Autodesk Inventor part; units mm, degrees
note: some values were not read from the file. Chosen so that the rebuilt part matches the saved one: direction of "Hole1"; direction of "Hole2".
(part 2 of 2)
sketch "Sketch23" plane through (-31.8897, 11.2835, 1.2) normal (0, 1, 0) x (1, 0, 0)
  spline S0 degree 3 poles (23.3423, 2.1773) (22.9361, 2.2868) (22.2348, 2.4758) (21.6643, 2.8122) (20.9702, 2.8356) (21.0959, 3.0801) (21.2357, 3.2556) (21.545, 3.6296) (22.0063, 4.1628) (22.2757, 4.6965) (22.7863, 5.1713) (22.4442, 5.3817) (22.141, 5.5963) (20.9793, 6.2853) (19.3097, 7.5226) (17.5595, 9.6465) (16.7918, 11.5742) (16.5566, 12.9888) (16.5569, 13.9187) (16.7809, 15.2775) (17.4991, 17.0874) (19.0032, 19.0617) (20.3636, 20.2269) (21.2697, 20.7719) (21.4294, 20.8993) (21.6261, 20.977) (21.4367, 21.2372) (21.2991, 21.56) (20.9903, 22.0433) (20.7038, 22.5269) (20.5306, 22.8626) (20.3527, 23.2142) (21.0187, 23.2936) (21.6089, 23.6536) (22.2816, 23.8828) (22.6704, 24.0153) knots 0 0 0 0 0.120251 0.207576 0.243092 0.253486 0.278932 0.314291 0.397791 0.481584 0.525055 0.542669 0.585382 0.644073 0.940951 1.209833 1.457149 1.553131 1.638804 1.734787 1.964951 2.214573 2.471025 2.502064 2.525764 2.536995 2.553986 2.597546 2.658422 2.719524 2.763708 2.781717 2.817624 2.904325 3.023078 3.023078 3.023078 3.023078
  line L0 (22.6704, 24.0153) -> (24.8571, 24.8395)
  line L1 (24.8571, 24.8395) -> (25.7117, 23.9446)
  line L2 (25.7117, 23.9446) -> (26.5664, 23.0497)
  line L3 (26.5664, 23.0497) -> (27.2264, 23.2249)
  spline S1 degree 3 poles (27.2264, 23.2249) (28.1214, 23.3942) (30.0601, 23.7608) (33.0033, 23.8407) (35.2391, 23.7446) (36.5812, 23.5025) (37.0345, 23.4774) (37.3791, 23.3665) (37.6145, 23.6266) (37.901, 23.9483) (38.2952, 24.4873) (38.6552, 24.9486) (38.9707, 25.3794) (39.3411, 25.3443) (39.7891, 25.1189) (40.555, 24.8644) (41.485, 24.483) (42.4572, 24.1727) (43.0299, 23.8169) (43.5284, 23.7887) (43.5573, 23.623) (43.5154, 23.5368) (43.3485, 23.2629) (42.9997, 22.7627) (42.8221, 22.2309) (42.3636, 21.7129) (42.6831, 21.5669) (42.9326, 21.3965) (43.4921, 21.0841) (44.2214, 20.6257) (45.0881, 20.0008) (45.6191, 19.5378) (45.8847, 19.3063) knots 0 0 0 0 0.27293 0.59117 0.879686 0.945407 0.996033 1.020616 1.042904 1.091245 1.155662 1.23829 1.276828 1.298799 1.342169 1.428477 1.539037 1.646645 1.725219 1.757766 1.763106 1.772735 1.785452 1.860503 1.945316 1.986613 2.00195 2.036474 2.082721 2.190949 2.296581 2.40228 2.40228 2.40228 2.40228
  line L4 (45.8847, 19.3063) -> (46.4831, 18.7637)
  line L5 (46.4831, 18.7637) -> (45.5703, 17.7587)
  spline S2 degree 3 poles (45.5703, 17.7587) (45.3819, 17.552) (44.9926, 17.1246) (44.4311, 16.5127) (44.0571, 16.1085) (43.8856, 15.9233) knots 0 0 0 0 0.336837 0.696095 1 1 1 1
  line L6 (43.8856, 15.9233) -> (43.1137, 15.0928)
  line L7 (43.1137, 15.0928) -> (42.5787, 15.6278)
  spline S3 degree 3 poles (42.5787, 15.6278) (42.3692, 15.8216) (41.9418, 16.2171) (41.4347, 16.5497) (40.7785, 17.1236) (40.7564, 16.0848) (40.6522, 15.2342) (40.6358, 13.8016) (40.695, 12.2687) (40.9149, 11.2921) (40.9213, 9.8853) (41.7084, 10.5187) (42.2359, 10.931) (42.7621, 11.4456) (43.0392, 11.7879) (43.1734, 11.9381) (43.6929, 12.1595) (44.4272, 10.4542) (45.2768, 9.6626) (46.909, 8.4425) (45.7357, 7.4784) (44.7926, 6.6607) (43.8619, 6.074) (43.3923, 5.7779) knots 0 0 0 0 0.082911 0.169166 0.215748 0.265595 0.383869 0.529269 0.678148 0.82545 0.902455 0.951972 1.051523 1.135634 1.163689 1.184755 1.195052 1.326968 1.555912 1.683629 1.767528 1.928068 2.091612 2.091612 2.091612 2.091612
  line L8 (43.3923, 5.7779) -> (42.7029, 5.3889)
  line L9 (42.7029, 5.3889) -> (43.1481, 4.5648)
  spline S4 degree 3 poles (43.1481, 4.5648) (43.2228, 4.4226) (43.352, 4.1771) (43.4776, 3.9019) (43.5917, 3.602) (42.9857, 3.4959) (42.4349, 3.0893) (41.808, 2.8165) (41.4455, 2.6589) knots 0 0 0 0 0.144061 0.248838 0.292599 0.397651 0.651775 1 1 1 1
  line L10 (41.4455, 2.6589) -> (39.4064, 1.6857)
  line L11 (39.4064, 1.6857) -> (38.497, 2.6351)
  line L12 (38.497, 2.6351) -> (37.5877, 3.5846)
  line L13 (37.5877, 3.5846) -> (36.7047, 3.4176)
  spline S5 degree 3 poles (36.7047, 3.4176) (35.8356, 3.3011) (34.0016, 3.0552) (31.2202, 3.0969) (29.1623, 3.2825) (27.933, 3.5282) (27.5632, 3.5571) (27.2655, 3.657) (27.0602, 3.3788) (26.7845, 3.0458) (26.4434, 2.5398) (26.1111, 2.0336) (25.8529, 1.7061) (25.644, 1.3775) (25.1343, 1.7051) (24.3983, 1.8109) (23.7297, 2.0429) (23.3423, 2.1773) knots 0 0 0 0 0.262808 0.554598 0.831023 0.884862 0.926436 0.946761 0.968531 1.017577 1.083667 1.149205 1.196727 1.216068 1.251541 1.338849 1.459095 1.459095 1.459095 1.459095
  spline S6 degree 3 poles (33.4664, 7.8872) (33.3675, 8.005) (33.0206, 8.4182) (32.2829, 9.1983) (31.2729, 10.2635) (30.2709, 11.3675) (29.3941, 12.1654) (29.0478, 12.723) (28.5693, 12.9441) (28.7979, 11.6512) (28.7224, 11.0547) (28.6664, 10.6128) knots 0 0 0 0 0.046143 0.161821 0.322037 0.485953 0.611319 0.670995 0.687359 0.74543 0.911379 0.911379 0.911379 0.911379
  line L14 (28.6664, 10.6128) -> (28.6664, 8.1986)
  line L15 (28.6664, 8.1986) -> (29.6564, 8.0671)
  spline S7 degree 3 poles (29.6564, 8.0671) (30.2463, 8.0061) (31.3137, 7.8959) (32.5931, 7.7585) (33.2683, 7.858) (33.4664, 7.8872) knots 0 0 0 0 0.465962 0.84327 1 1 1 1
  spline S8 degree 3 poles (24.346, 11.5638) (24.3332, 12.0912) (24.3084, 13.1122) (24.1246, 14.5806) (23.8837, 15.498) (23.7683, 15.9376) knots 0 0 0 0 0.35758 0.692157 1 1 1 1
  line L16 (23.7683, 15.9376) -> (23.5562, 16.6338)
  line L17 (23.5562, 16.6338) -> (22.8911, 16.0051)
  spline S9 degree 3 poles (22.8911, 16.0051) (22.4328, 15.5195) (21.6033, 14.6409) (21.4421, 12.707) (22.2632, 11.4954) (23.1271, 10.6526) (23.6304, 10.3409) (24.1516, 9.8404) (24.3516, 10.2378) (24.3172, 10.763) (24.3346, 11.2475) (24.346, 11.5638) knots 0 0 0 0 0.195516 0.353825 0.536032 0.620113 0.701515 0.748907 0.76593 0.816085 0.910347 0.910347 0.910347 0.910347
  spline S10 degree 3 poles (35.823, 18.6972) (35.6212, 18.7497) (35.0066, 18.9098) (33.834, 18.9362) (32.8792, 18.9436) (32.3496, 18.9477) knots 0 0 0 0 0.17869 0.544357 1 1 1 1
  line L18 (32.3496, 18.9477) -> (30.4528, 18.9138)
  line L19 (30.4528, 18.9138) -> (33.1296, 16.0653)
  line L20 (33.1296, 16.0653) -> (35.8064, 13.2168)
  line L21 (35.8064, 13.2168) -> (35.8387, 15.933)
  spline S11 degree 3 poles (35.8387, 15.933) (35.8415, 16.3912) (35.8463, 17.1803) (35.8565, 18.1024) (35.8304, 18.5651) (35.823, 18.6972) knots 0 0 0 0 0.497248 0.856443 1 1 1 1
  point P0 (22.1954, 2.5387)
  point P1 (21.365, 2.8089)
  point P2 (21.0309, 2.9293)
  point P3 (21.07, 3.0256)
  point P4 (21.2181, 3.2325)
  point P5 (21.4432, 3.5052)
  point P6 (21.964, 4.1579)
  point P7 (22.4511, 4.8397)
  point P8 (22.6664, 5.2173)
  point P9 (22.5308, 5.3297)
  point P10 (22.1751, 5.5662)
  point P11 (21.6764, 5.8757)
  point P12 (19.316, 7.6763)
  point P13 (17.6389, 9.778)
  point P14 (16.7278, 12.0772)
  point P15 (16.5788, 13.0254)
  point P16 (16.5788, 13.8821)
  point P17 (16.7278, 14.8303)
  point P18 (17.5627, 16.9752)
  point P19 (19.0495, 18.9803)
  point P20 (21.0212, 20.6202)
  point P21 (21.2824, 20.7879)
  point P22 (21.4816, 20.9164)
  point P23 (21.5755, 20.9779)
  point P24 (21.514, 21.1363)
  point P25 (21.3054, 21.5187)
  point P26 (20.995, 22.0424)
  point P27 (20.686, 22.5695)
  point P28 (20.481, 22.9609)
  point P29 (20.4245, 23.1319)
  point P30 (20.754, 23.2747)
  point P31 (21.5609, 23.592)
  point P32 (29.9198, 23.666)
  point P33 (33.0992, 23.8044)
  point P34 (35.9776, 23.6058)
  point P35 (36.6276, 23.5091)
  point P36 (37.1291, 23.4401)
  point P37 (37.3736, 23.4138)
  point P38 (37.5476, 23.553)
  point P39 (37.8648, 23.9178)
  point P40 (38.2563, 24.4293)
  point P41 (38.7556, 25.0877)
  point P42 (39.0406, 25.3471)
  point P43 (39.2603, 25.3431)
  point P44 (39.6657, 25.189)
  point P45 (40.4726, 24.8828)
  point P46 (41.5064, 24.4909)
  point P47 (42.5114, 24.1062)
  point P48 (43.2428, 23.819)
  point P49 (43.5422, 23.6914)
  point P50 (43.5506, 23.6387)
  point P51 (43.5192, 23.5476)
  point P52 (43.4547, 23.438)
  point P53 (43.0595, 22.8)
  point P54 (42.6491, 22.0578)
  point P55 (42.4826, 21.6799)
  point P56 (42.6116, 21.5968)
  point P57 (42.9075, 21.4191)
  point P58 (43.3064, 21.185)
  point P59 (44.2236, 20.6106)
  point P60 (45.0774, 19.9885)
  point P61 (45.0048, 17.1387)
  point P62 (44.3995, 16.4793)
  point P63 (41.9574, 16.1769)
  point P64 (41.2719, 16.7004)
  point P65 (40.8688, 16.9338)
  point P66 (40.7601, 16.4473)
  point P67 (40.6768, 15.2675)
  point P68 (40.6485, 13.8138)
  point P69 (40.7293, 12.3272)
  point P70 (40.9016, 10.8643)
  point P71 (41.084, 10.1162)
  point P72 (41.5142, 10.3615)
  point P73 (42.2829, 10.994)
  point P74 (42.8758, 11.5906)
  point P75 (43.0566, 11.8052)
  point P76 (43.2108, 11.9487)
  point P77 (43.305, 11.9901)
  point P78 (44.2237, 11.0435)
  point P79 (45.7418, 9.3297)
  point P80 (46.5428, 8.3349)
  point P81 (46.0015, 7.6938)
  point P82 (44.755, 6.6821)
  point P83 (43.3649, 4.1422)
  point P84 (43.5053, 3.8266)
  point P85 (43.5389, 3.6863)
  point P86 (43.2322, 3.5256)
  point P87 (42.4801, 3.1565)
  point P88 (34.0925, 3.1295)
  point P89 (31.1746, 3.1348)
  point P90 (28.4264, 3.4327)
  point P91 (27.8958, 3.5238)
  point P92 (27.4852, 3.5888)
  point P93 (27.2834, 3.6136)
  point P94 (27.1232, 3.4662)
  point P95 (26.8215, 3.0796)
  point P96 (26.4434, 2.5375)
  point P97 (26.0741, 1.9961)
  point P98 (25.7949, 1.6115)
  point P99 (25.6664, 1.4669)
  point P100 (25.3259, 1.5664)
  point P101 (24.491, 1.8216)
  point P102 (33.1677, 8.2389)
  point P103 (32.3847, 9.0904)
  point P104 (31.2868, 10.2572)
  point P105 (30.1587, 11.4464)
  point P106 (29.2964, 12.3565)
  point P107 (28.8868, 12.7904)
  point P108 (28.7344, 12.8501)
  point P109 (28.6759, 12.2723)
  point P110 (31.4294, 7.8826)
  point P111 (32.8713, 7.8145)
  point P112 (24.2803, 13.1449)
  point P113 (24.0864, 14.6128)
  point P114 (21.7368, 14.427)
  point P115 (21.6137, 12.8487)
  point P116 (22.5216, 11.2689)
  point P117 (23.1286, 10.6871)
  point P118 (23.7731, 10.1899)
  point P119 (24.1964, 9.9768)
  point P120 (24.2853, 10.1219)
  point P121 (24.3324, 10.6213)
  point P122 (35.2151, 18.8391)
  point P123 (33.9411, 18.931)
  point P124 (35.8484, 17.3077)
  point P125 (35.8428, 18.3008)
  point P126 (35.8387, 15.933)
  point P127 (35.8064, 13.2168)
  point P128 (33.1296, 16.0653)
  point P129 (35.823, 18.6972)
  point P130 (23.7683, 15.9376)
  point P131 (24.346, 11.5638)
  point P132 (22.8911, 16.0051)
  constraints: 44 end point, 150 other
extrude "Extrusion9" cut sketch "Sketch23" against normal blind 1 keep common part
pattern_circular "Circular Pattern2" count 2 over 360 about axis through (0, 0, -25.977) along (0, 0, -1)
split body "Split6" result two bodies by plane through (0, 0, 0) normal (0, 1, 0) first body at (5.4592, 10.7835, -6.0203)
sketch "Sketch17" plane through (-27.1085, -2.321, -21.5638) normal (0, 1, 0) x (1, 0, 0)
  line L0 (0, 0) -> (3.9034, 0) projected
  line L1 (3.9034, 0) -> (3.9034, 4.4131) projected
  line L2 (3.9034, 4.4131) -> (0, 4.4131) projected
  line L3 (0, 4.4131) -> (0, 0) projected
  line L4 (0, 4.4131) -> (0, 0) projected
  line L5 (3.9034, 0) -> (0, 4.4131)
  circle A0 centre (1.9517, 2.2066) radius 0.6
  point P0 (27.1085, -21.5638)
  dimension "d84" = 1.2
  constraints: 2 end point, 1 centre point, 1 midpoint
  measures "d84" diameter of A0
sketch "Sketch18" plane through (23.205, 2.3119, -25.977) normal (0, -1, 0) x (1, 0, 0)
  line L0 (0, 4.4131) -> (0, 0) projected
  line L1 (0, 0) -> (3.9034, 0) projected
  line L2 (3.9034, 0) -> (3.9034, 4.4131) projected
  line L3 (3.9034, 4.4131) -> (0, 4.4131) projected
  line L4 (3.9034, 4.4131) -> (0, 4.4131) projected
  line L5 (0, 0) -> (3.9034, 4.4131)
  circle A0 centre (1.9517, 2.2066) radius 0.6
  point P0 (-23.205, 25.977)
  dimension "d87" = 1.2
  constraints: 2 end point, 1 centre point, 1 midpoint
  measures "d87" diameter of A0
sketch "Sketch19" plane through (-27.1085, -2.321, -21.5638) normal (0, -1, 0) x (1, 0, 0)
  line L0 (0, -4.4131) -> (0, 0) projected
  line L1 (0, 0) -> (3.9034, -4.4131)
  point P0 (27.1085, 21.5638)
  point P1 (1.9517, -2.2066)
  constraints: 2 end point, 1 coincident, 1 midpoint
sketch "Sketch20" plane through (23.205, 2.3119, -21.5638) normal (0, 1, 0) x (1, 0, 0)
  line L0 (0, 4.4131) -> (0, 0) projected
  line L1 (-46.4101, 0) -> (3.9034, 0) projected
  line L2 (0, 4.4131) -> (3.9034, 0)
  point P0 (-23.205, -21.5638)
  point P1 (3.3532, 0)
  point P2 (1.9517, 2.2066)
  constraints: 2 end point, 1 midpoint
body "Srf3"
body "Solid8"
body "Solid9"
body "Solid10"
body "Solid11"
body "Solid12"
body "Solid13"
